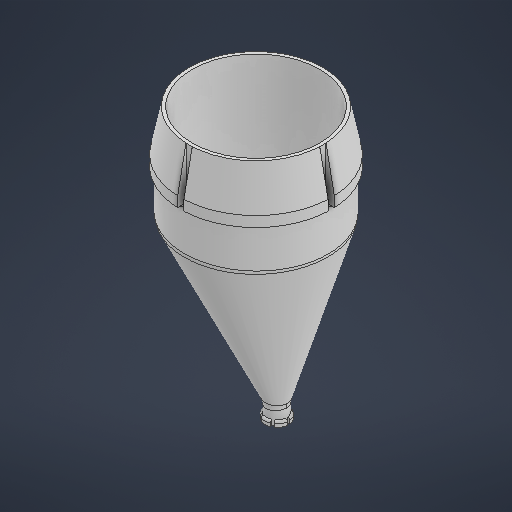
# Autodesk Inventor part: SACMI PH1500 HOPPER
Saved by Autodesk Inventor 2025 (Build 290162000, 162)
## iProperties
Created: 2024-05-05
Part Number: SACMI PH1500 HOPPER
Material: Generic
Document SubType Name: Modeling
Designer: zulet
Density: 1 g/cm^3
Appearance: Default
Author: zulet
Autodesk Inventor part; units mm, degrees
ref_plane "YZ Plane" through (0, 0, 0) normal (1, 0, 0) x (0, 1, 0)
ref_plane "XZ Plane" through (0, 0, 0) normal (0, 1, 0) x (-1, 0, 0)
ref_plane "XY Plane" through (0, 0, 0) normal (0, 0, 1) x (1, 0, 0)
sketch "Sketch1" plane through (0, 0, 0) normal (0, 1, 0) x (-1, 0, 0)
  circle A0 centre (0, 0) radius 695
  circle A1 centre (0, 0) radius 615
  dimension "d0" = 1390
  dimension "d30" = 80
  constraints: 2 centre point, 1 coincident
  measures "d0" diameter of A0
  measures "d30" radial gap between concentric circles of A0 A1
extrude "Extrusion1" add sketch "Sketch1" along normal blind 400 contours A0 | A1
sketch "Sketch2" plane through (0, 400, 0) normal (0, 1, 0) x (1, 0, 0)
  circle A0 centre (0, 0) radius 695 projected
  circle A1 centre (0, 0) radius 725
  circle A2 centre (0, 0) radius 615 projected
  dimension "d3" = 30
  constraints: 1 centre point
  measures "d3" radial gap between concentric circles of A0 A1
extrude "Extrusion2" add sketch "Sketch2" along normal blind 500 contours A0 | A1
chamfer "Chamfer1" distance 80 distance2 400 1 edges at (-725, 900, 0) measured on face at (-724.5, 900, 0)
sketch "Sketch3" plane through (0, 900, 0) normal (0, 1, 0) x (1, 0, 0)
  line L0 (800, 30) -> (-800, 30)
  line L1 (-800, 30) -> (-800, -30)
  line L2 (-800, -30) -> (800, -30)
  line L3 (800, -30) -> (800, 30)
  line L4 (800, 30) -> (-800, -30) construction
  line L5 (-800, 30) -> (800, -30) construction
  line L6 (30, 800) -> (-30, 800)
  line L7 (-30, 800) -> (-30, -800)
  line L8 (-30, -800) -> (30, -800)
  line L9 (30, -800) -> (30, 800)
  line L10 (30, 800) -> (-30, -800) construction
  line L11 (-30, 800) -> (30, -800) construction
  circle A0 centre (0, 0) radius 645 projected
  point P0 (30, -644.3019)
  point P1 (-30, -644.3019)
  point P2 (644.3019, 30)
  point P3 (644.3019, -30)
  point P4 (-30, 644.3019)
  point P5 (30, 644.3019)
  point P6 (-644.3019, -30)
  point P7 (-644.3019, 30)
  dimension "d9" = 1600
  dimension "d10" = 60
  dimension "d11" = 60
  dimension "d12" = 1600
  constraints: 24 end point, 4 midpoint, 4 parallel, 2 horizontal, 2 perpendicular
  measures "d9" distance of L2.end L1.end
  measures "d10" distance of L1.end L0.end
  measures "d11" distance of L8.end L7.end
  measures "d12" distance of L7.end L6.end
extrude "Extrusion3" cut sketch "Sketch3" against normal up to surface (500 mm away) contours L3 L2 A0 L0 | A0 L7 L6 L9 | L9 L8 L7 A0 | A0 L2 L1 L0
ref_plane "Work Plane1" through (0, -1600, 0) normal (0, -1, 0) x (1, 0, 0)
sketch "Sketch4" plane through (0, -1600, 0) normal (0, -1, 0) x (1, 0, 0)
  circle A0 centre (200, 0) radius 95
  line L0 (0, 0) -> (200, 0) construction
  circle A1 centre (200, 0) radius 115
  line L1 (105.826, 12.5) -> (85.6814, 12.5)
  line L2 (105.826, -12.5) -> (85.6814, -12.5)
  line L3 (142.0877, -75.3071) -> (132.0154, -92.7528)
  line L4 (163.7383, -87.8071) -> (153.666, -105.2528)
  line L5 (236.2617, -87.8071) -> (246.334, -105.2528)
  line L6 (257.9123, -75.3071) -> (267.9846, -92.7528)
  line L7 (294.174, -12.5) -> (314.3186, -12.5)
  line L8 (294.174, 12.5) -> (314.3186, 12.5)
  line L9 (257.9123, 75.3071) -> (267.9846, 92.7528)
  line L10 (236.2617, 87.8071) -> (246.334, 105.2528)
  line L11 (163.7383, 87.8071) -> (153.666, 105.2528)
  line L12 (142.0877, 75.3071) -> (132.0154, 92.7528)
  circle A2 centre (200, 0) radius 70
  dimension "d16" = 190
  dimension "d20" = 20
  dimension "d17" = 200
  dimension "d21" = 25
  dimension "d24" = 360
  dimension "d29" = 25
  constraints: 26 end point, 2 horizontal, 2 symmetric about line, 1 centre point, 43 other
  measures "d17" distance of L0.start L0.end
  measures "d21" distance between parallel lines of L2 L1
extrude "Extrusion4" add sketch "Sketch4" against normal blind 150 contours A0 | A2
extrude "Extrusion5" add sketch "Sketch4" against normal blind 50 contours A0 L9 A1 L8 | L7 A1 L6 A0 | A0 L11 A1 L10 | L5 A1 L4 A0 | A0 L1 A1 L12 | L3 A1 L2 A0
fillet "Fillet1" radius 20 6 edges at (100.4071, -1550, -57.5) (100.4071, -1550, 57.5) (200, -1550, 115) (299.5929, -1550, 57.5) (299.5929, -1550, -57.5) (200, -1550, -115)
sketch "Sketch5" plane through (200, -1450, 0) normal (0, 1, 0) x (1, 0, 0)
  circle A0 centre (0, 0) radius 95 projected
  line L0 (0, 0) -> (95, 0) construction
  point P0 (-200, 0)
  point P1 (47.5, 82.2724)
  point P2 (-47.5, 82.2724)
  point P3 (-95, 0)
  point P4 (-47.5, -82.2724)
  point P5 (47.5, -82.2724)
  dimension "d33" = 360
  constraints: 2 end point, 1 horizontal, 1 horizontal alignment, 8 other
sketch "Sketch6" plane through (0, 0, 0) normal (0, -1, 0) x (1, 0, 0)
  circle A0 centre (0, 0) radius 695 projected
  line L0 (0, 0) -> (695, 0) construction
  point P0 (347.5, 601.8877)
  point P1 (-347.5, 601.8877)
  point P2 (-695, 0)
  point P3 (-347.5, -601.8877)
  point P4 (347.5, -601.8877)
  dimension "d37" = 360
  constraints: 2 end point, 1 coincident, 1 horizontal, 1 horizontal alignment, 8 other
sketch3d "3D Sketch1"
loft "Loft1" add section 1 edges at (695, 0, 0) section 2 edges at (105, -1450, 0)
sketch "Sketch7" plane through (0, 400, 0) normal (0, 1, 0) x (1, 0, 0)
  circle A0 centre (0, 0) radius 615 projected
extrude "Extrusion6" cut sketch "Sketch7" against normal blind 400
sketch "Sketch8" plane through (0, -1600, 0) normal (0, -1, 0) x (1, 0, 0)
  circle A0 centre (200, 0) radius 95 projected
  circle A1 centre (200, 0) radius 70
  point P0 (0, 0)
  dimension "d45" = 25
  constraints: 1 centre point
  measures "d45" radial gap between concentric circles of A0 A1
extrude "Extrusion7" cut sketch "Sketch8" against normal blind 150 contours A1
loft "Loft2" cut section 1 edges at (-615, 0, 0) section 2 edges at (130, -1450, 0)
fillet "Fillet2" radius 100 2 edges at (0, 0, 695) (0, 0, -695)
fillet "Fillet3" radius 150 2 edges at (200, -1450, 95) (200, -1450, -95)
body "Solid1"
